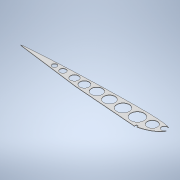
# Autodesk Inventor part: airfoil
Saved by Autodesk Inventor 2022 (Build 260153000, 153)
## iProperties
Created: 2021-03-06
Part Number: airfoil
Material: Generic
Document SubType Name: Modeling
Designer: Ferdinand Hubbard
Density: 1 g/cm^3
Appearance: Default
Author: Ferdinand Hubbard
Autodesk Inventor part; units mm, degrees
ref_plane "YZ Plane" through (0, 0, 0) normal (1, 0, 0) x (0, 1, 0)
ref_plane "XZ Plane" through (0, 0, 0) normal (0, 1, 0) x (-1, 0, 0)
ref_plane "XY Plane" through (0, 0, 0) normal (0, 0, 1) x (1, 0, 0)
sketch "Sketch1" plane through (0, 0, 0) normal (0, 1, 0) x (-1, 0, 0)
  line L0 (211.4974, 21.8387) -> (51.979, 34.2431)
  line L1 (362.8741, 0.9685) -> (367.8741, 0.9685)
  line L2 (367.8741, 0.9685) -> (367.8741, -4.0315)
  line L3 (367.8741, -4.0315) -> (362.8741, -4.0315)
  line L4 (362.8741, -4.0315) -> (362.8741, 0.9685)
  line L5 (211.4974, 21.8387) -> (210.0997, -8.5616) construction
  line L6 (46.4065, 34.5291) -> (51.4065, 34.5291)
  line L7 (51.4065, 34.5291) -> (51.4065, 29.5291)
  line L8 (51.4065, 29.5291) -> (46.4065, 29.5291)
  line L9 (46.4065, 29.5291) -> (46.4065, 34.5291)
  line L10 (46.4065, 34.5291) -> (51.4065, 29.5291) construction
  line L11 (51.4065, 34.5291) -> (46.4065, 29.5291) construction
  circle A0 centre (8.4978, 2.2571) radius 7.5
  circle A1 centre (139.6638, 8.2367) radius 14
  circle A2 centre (104.507, 9.4908) radius 15.5
  circle A3 centre (172.721, 6.5051) radius 13.5
  circle A4 centre (259.3726, 4.4053) radius 7.5
  circle A5 centre (67.3244, 10.9193) radius 16.5
  circle A6 centre (203.331, 6.9819) radius 11.5
  circle A7 centre (229.7182, 5.2903) radius 10
  line L12 (1.6385, 5.2903) -> (2.3233, 7.7402)
  line L13 (5.9301, -4.7897) -> (7.0011, -5.598)
  spline S0 degree 4 poles (51.979, 34.2431) (49.1051, 33.7566) (39.5332, 31.5872) (30.1137, 28.1904) (19.6059, 22.8943) (13.0923, 18.5073) (7.8605, 14.3051) (4.5473, 10.1712) (2.863, 8.0733) (2.0995, 6.7311) (1.9781, 6.5051) knots 0 0 0 0 0 0.341108 0.484452 0.62044 0.748582 0.868222 0.978476 1 1 1 1 1
  spline S1 degree 4 poles (6.5182, -5.2336) (7.9483, -5.7218) (11.6839, -6.8944) (16.0214, -7.493) (25.5133, -9.1262) (35.8155, -9.8616) (48.4495, -10.5455) (62.4279, -10.8762) (77.9663, -11.0677) (94.722, -11.0635) (112.5613, -10.9225) (131.2432, -10.6462) (150.5553, -10.2615) (170.2642, -9.7779) (190.1377, -9.2151) (209.9398, -8.5807) (229.4366, -7.8911) (248.3971, -7.1484) (266.6047, -6.3637) (283.8414, -5.5226) (299.9482, -4.5961) (314.7433, -3.6129) (328.1612, -2.6484) (339.8268, -1.769) (350.012, -1.0496) (357.5866, -0.5225) (364.806, -0.1794) (367.4848, -0.031) (370.1657, -0.0078) (369.9872, 0.0018) knots 0.255434 0.255434 0.255434 0.255434 0.255434 0.272366 0.294434 0.318911 0.345468 0.373865 0.403873 0.435249 0.467749 0.501146 0.535218 0.569752 0.604537 0.639365 0.674029 0.708317 0.742021 0.774934 0.806859 0.837599 0.866942 0.894636 0.920358 0.943684 0.964014 0.980302 1 1 1 1 1
  line L14 (5.0928, 12.3024) -> (-1.1366, 0.7079) construction
  arc A8 (5.0901, 10.4454) -> (0.4104, 1.7352) centre (14.6462, -0.301) ccw construction
  line L15 (-27.4852, 6.3739) -> (40.5216, -16.8411) construction
  arc A9 (-17.1067, 8.2367) -> (33.4484, -9.0209) centre (29.8704, 63.1753) ccw construction
  circle A10 centre (32.7718, 8.2367) radius 12.5
  circle A11 centre (281.2667, 3.3987) radius 6
  line L16 (211.4974, 21.8387) -> (370.1606, 1.1994)
  circle A12 centre (370.1606, 1.1994) radius 4 construction
  line L17 (367.8741, 0.9685) -> (366.8087, 1.6354)
  point P0 (0, 0)
  point P1 (370, 0)
  point P2 (35.937, 30.0257)
  point P3 (27.0238, 26.4761)
  point P4 (19.2974, 22.4624)
  point P5 (12.8156, 18.139)
  point P6 (7.6237, 13.6489)
  point P7 (3.7499, 9.1521)
  point P8 (1.2115, 4.8535)
  point P9 (0.0668, 1.0195)
  point P10 (0.0003, -0.0638)
  point P11 (0.0755, -0.9849)
  point P12 (0.2106, -1.5356)
  point P13 (0.4302, -2.0122)
  point P14 (0.7739, -2.4345)
  point P15 (1.2488, -2.8423)
  point P16 (2.1566, -3.4383)
  point P17 (3.2773, -4.0196)
  point P18 (15.3669, -7.4261)
  point P19 (24.3167, -8.7706)
  point P20 (35.0526, -9.7678)
  point P21 (47.5438, -10.4262)
  point P22 (61.6814, -10.8267)
  point P23 (77.2847, -11.0213)
  point P24 (94.162, -11.0379)
  point P25 (112.1091, -10.9014)
  point P26 (130.911, -10.6315)
  point P27 (150.3435, -10.2474)
  point P28 (170.176, -9.7646)
  point P29 (190.1737, -9.1986)
  point P30 (229.7182, -7.8653)
  point P31 (248.7963, -7.1166)
  point P32 (267.1071, -6.3194)
  point P33 (284.4371, -5.4606)
  point P34 (300.619, -4.5258)
  point P35 (315.5184, -3.5432)
  point P36 (328.988, -2.5786)
  point P37 (340.8625, -1.7041)
  point P38 (350.9622, -0.9861)
  point P39 (359.0984, -0.4682)
  point P40 (365.0855, -0.1602)
  point P41 (368.7597, -0.0285)
  point P42 (369.9872, 0.0018)
  point P43 (48.9065, 32.0291)
  point P44 (112.1091, -11.9485)
  point P45 (1.9781, 6.5051)
  point P46 (51.4065, 34.1414)
  point P47 (46.4065, 33.0501)
  point P48 (362.8741, -0.2698)
  point P49 (367.8741, -0.0505)
  dimension "d8" = 160
  dimension "d26" = 5
  dimension "d27" = 5
  dimension "d36" = 5
  dimension "d37" = 5
  dimension "d50" = 368.7594
  dimension "d51" = 15
  dimension "d52" = 28
  dimension "d53" = 31
  dimension "d54" = 27
  dimension "d57" = 15
  dimension "d59" = 33
  dimension "d61" = 23
  dimension "d62" = 20
  dimension "d65" = 44.6693
  dimension "d66" = 25
  dimension "d67" = 12
  dimension "d68" = 160
  dimension "d69" = 8
  constraints: 36 end point, 13 centre point, 6 midpoint, 4 parallel, 4 point on circle, 3 point on line, 2 horizontal, 2 perpendicular, 1 coincident, 42 other
  measures "d8" distance of L0.start L0.end
  measures "d26" distance of L2.end L3.end
  measures "d27" distance of L1.end L2.end
  measures "d36" distance of L7.end L8.end
  measures "d37" distance of L6.end L7.end
  measures "d50" distance of point (368.76, -0.028) point (0, -0.064)
  measures "d51" diameter of A0
  measures "d52" diameter of A1
  measures "d53" diameter of A2
  measures "d54" diameter of A3
  measures "d57" diameter of A4
  measures "d59" diameter of A5
  measures "d61" diameter of A6
  measures "d62" diameter of A7
  measures "d65" vertical distance of point (47.544, -10.426) L0.end
  measures "d66" diameter of A10
  measures "d67" diameter of A11
  measures "d68" distance of L0.start L16.end
  measures "d69" diameter of A12
extrude "Extrusion4" add sketch "Sketch1" along normal blind 1 contours L16 L17 L1 L4 S1 L13 A0 L12 S0 L9 L8 L7 L0
body "Solid4"
